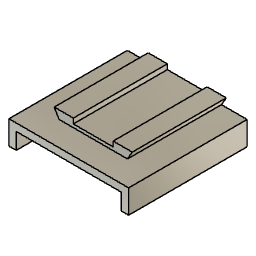
Dovetail_to_specs v2 (Autodesk Fusion 360 design; units mm, degrees)
Autodesk Fusion 360 part; units mm, degrees
sketch "Sketch1" plane through (0, 0, 0) normal (0, 0, 1) x (1, 0, 0)
  line L0 (0, 0) -> (4.8, 0)
  line L1 (4.8, 0) -> (4.8, 7.255)
  line L2 (4.8, 7.255) -> (0, 7.255)
  line L3 (0, 7.255) -> (0, 0)
  line L4 (0.3045, 7.255) -> (4.4955, 7.255)
  line L5 (4.4955, 7.255) -> (4.4955, 1.5)
  line L6 (4.4955, 1.5) -> (0.3045, 1.5)
  line L7 (0.3045, 1.5) -> (0.3045, 7.255)
  line L8 (1.181, 7.255) -> (3.619, 7.255)
  line L9 (3.619, 7.255) -> (3.619, 1.5)
  line L10 (3.619, 1.5) -> (1.181, 1.5)
  line L11 (1.181, 1.5) -> (1.181, 7.255)
  line L12 (2.4, 1.5) -> (2.4, 0) construction
  dimension "d1" = 7.255
  dimension "d2" = 4.8
  dimension "d3" = 5.755
  dimension "d4" = 4.191
  dimension "d5" = 2.438
  constraint horizontal L0
  constraint vertical L1
  constraint horizontal L2
  constraint vertical L3
  constraint coincident L0.start L3.end
  constraint horizontal L4
  constraint vertical L5
  constraint horizontal L6
  constraint vertical L7
  constraint coincident L2 L4.start
  constraint horizontal L8
  constraint vertical L9
  constraint horizontal L10
  constraint vertical L11
  constraint coincident L6 L9.end
  constraint coincident L2 L8.start
  constraint coincident L0 L12.end
  constraint perpendicular L0 L12
  constraint midpoint L0 L12.end
  constraint coincident L6 L12.start
  constraint midpoint L6 L12.start
  constraint midpoint L10 L12.start
  measures "d1" distance of L0.end L1.end
  measures "d2" distance of L0.start L0.end
  measures "d3" distance of L4.end L5.end
  measures "d4" distance of L5.end L6.end
  measures "d5" distance of L9.end L10.end
extrude "Extrude1" add sketch "Sketch1" along normal blind 0.45 contours L0 L1 L2 L3 L5 L6 L7 L10 makes body 1
extrude "Extrude2" add sketch "Sketch1" along normal blind 0.65 contours L2 L4 L6 L8 L9 L10 L11 bodies 1
extrude "Extrude3" add sketch "Sketch1" along normal blind 0.45 separate body contours L2 L4 L6 L7 L11 | L2 L4 L5 L6 L9 makes body 2 at (4.2033, 3.4183, 0) makes body 3 at (0.8888, 3.4183, 0)
extrude "Extrude4" add 1 faces at (0.8888, 3.4183, 0.45) along direction (0, 0, 1) blind 0.508 on bodies 3 bodies 3 2 1
sketch "Sketch2" plane through (0, 0, 0.45) normal (0, 0, 1) x (-1, 0, 0)
  line L0 (-4.4955, -1.5) -> (-3.619, -1.5)
  line L1 (-3.619, -1.5) -> (-0.3045, -1.5)
  line L2 (-0.3045, -1.5) -> (-0.3045, -7.255)
  line L3 (-0.3045, -7.255) -> (0, -7.255)
  line L4 (0, -7.255) -> (0, 0)
  line L5 (0, 0) -> (-4.8, 0)
  line L6 (-4.8, 0) -> (-4.8, -7.255)
  line L7 (-4.8, -7.255) -> (-4.4955, -7.255)
  line L8 (-4.4955, -7.255) -> (-4.4955, -1.5)
draft "Draft1" angle -30 neutral plane through (0, 0, 0.45) pull (0, 0, 1) 1 faces at (0.3045, 5.3367, 0.6193) on bodies 3
extrude "Extrude5" add 1 faces at (4.2033, 3.4183, 0.45) along direction (0, 0, 1) blind 0.508 on bodies 2 bodies 2 3
draft "Draft2" angle -30 neutral plane through (0, 0, 0.45) pull (0, 0, 1) 1 faces at (4.4955, 3.4183, 0.7887) on bodies 2
copy_body "Body->Comp1" bodies 2 removing the originals makes body 4 in component "Component"
move_face "OffsetFaces1" offset 0.815 1 faces at (4.8, 4.8367, 0.3) on bodies 4 in component "Component"
move_face "OffsetFaces2" offset 0.815 1 faces at (0, 4.8367, 0.15) on bodies 4 in component "Component"
sketch "Sketch3" plane through (0, 0, 0.45) normal (0, 0, 1) x (-1, 0, 0)
  line L0 (-4.4955, -1.5) -> (-0.3045, -1.5)
  line L1 (-0.3045, -1.5) -> (-0.3045, -7.255)
  line L2 (-0.3045, -7.255) -> (0.815, -7.255)
  line L3 (0.815, -7.255) -> (0.815, 0)
  line L4 (0.815, 0) -> (-5.615, 0)
  line L5 (-5.615, 0) -> (-5.615, -7.255)
  line L6 (-5.615, -7.255) -> (-4.4955, -7.255)
  line L7 (-4.4955, -7.255) -> (-4.4955, -1.5)
  line L8 (0.815, 0) -> (1.265, 0)
  line L9 (1.265, 0) -> (1.265, -7.255)
  line L10 (1.265, -7.255) -> (0.815, -7.255)
  line L11 (0.815, -7.255) -> (0.815, 0)
  line L12 (-5.615, -7.255) -> (-6.065, -7.255)
  line L13 (-6.065, -7.255) -> (-6.065, 0)
  line L14 (-6.065, 0) -> (-5.615, 0)
  line L15 (-5.615, 0) -> (-5.615, -7.255)
  dimension "d22" = 0.45
  dimension "d23" = 0.45
  constraint horizontal L8
  constraint vertical L9
  constraint horizontal L10
  constraint vertical L11
  constraint coincident L3.end L4.start
  constraint horizontal L12
  constraint vertical L13
  constraint horizontal L14
  constraint vertical L15
  constraint coincident L5.end L6.start
  measures "d22" distance of L9.end L2.end
  measures "d23" distance of L5.end L12.end
extrude "Extrude2'" add sketch "Sketch3" against normal blind 1.45 contours L3 L8 L9 L10 L11 bodies 4 in component "Component"
extrude "Extrude1'" add sketch "Sketch3" against normal blind 1.45 contours L5 L12 L13 L14 L15 bodies 4 in component "Component"
component "Component" placed x (1, 0, 0) y (0, 1, 0) z (0, 0, 1) at (0, 0, 0)
